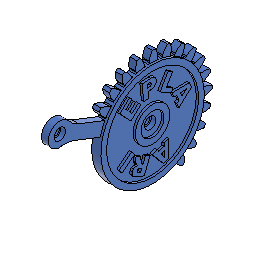
05 Engranaje grande superior (Autodesk Fusion 360 design; units mm, degrees)
Autodesk Fusion 360 part; units mm, degrees
(part 1 of 6)
sketch "Boceto1" plane through (0, 0, 0) normal (0, 0, 1) x (1, 0, 0)
  circle A0 centre (0, 0) radius 22.5
  circle A1 centre (0, 0) radius 0.5
extrude "Extruir1" add sketch "Boceto1" along normal blind 3
sketch "Boceto2" plane through (0, 0, 0) normal (0, 0, 1) x (1, 0, 0)
  spline S0 degree 5 poles (23.4214, -1.8244) (23.4316, -1.8252) (23.4521, -1.8265) (23.4829, -1.8277) (23.524, -1.8279) (23.5754, -1.8262) (23.6269, -1.8231) (23.6784, -1.819) (23.7299, -1.8145) (23.7814, -1.8097) (23.833, -1.8045) (23.8845, -1.7988) (23.9361, -1.7926) (23.9876, -1.7857) (24.0392, -1.7781) (24.0907, -1.7698) (24.1423, -1.761) (24.1939, -1.7518) (24.2454, -1.7421) (24.2969, -1.7321) (24.3485, -1.7216) (24.4, -1.7108) (24.4515, -1.6996) (24.503, -1.6879) (24.5544, -1.6758) (24.6059, -1.6633) (24.6573, -1.6504) (24.7087, -1.6371) (24.7602, -1.6235) (24.8115, -1.6095) (24.8629, -1.5952) (24.9142, -1.5805) (24.9655, -1.5655) (25.0168, -1.5501) (25.0681, -1.5344) (25.1193, -1.5184) (25.1706, -1.502) (25.2217, -1.4853) (25.2729, -1.4683) (25.324, -1.451) (25.3751, -1.4333) (25.4262, -1.4154) (25.4772, -1.3971) (25.5282, -1.3786) (25.5792, -1.3597) (25.6301, -1.3406) (25.6811, -1.3211) (25.7319, -1.3014) (25.7828, -1.2814) (25.8336, -1.2611) (25.8843, -1.2405) (25.935, -1.2196) (25.9857, -1.1985) (26.0364, -1.177) (26.087, -1.1553) (26.1375, -1.1334) (26.1881, -1.1111) (26.2386, -1.0886) (26.289, -1.0658) (26.3394, -1.0428) (26.3897, -1.0194) (26.4401, -0.9959) (26.4903, -0.972) (26.5405, -0.948) (26.5907, -0.9236) (26.6409, -0.899) (26.6909, -0.8742) (26.741, -0.849) (26.791, -0.8237) (26.8409, -0.7981) (26.8908, -0.7722) (26.9307, -0.7514) (26.9605, -0.7356) (26.9805, -0.725) (26.9904, -0.7197) knots 0 0 0 0 0 0 0.01428571 0.02857143 0.04285714 0.05714286 0.07142857 0.08571429 0.1 0.11428571 0.12857143 0.14285714 0.15714286 0.17142857 0.18571429 0.2 0.21428571 0.22857143 0.24285714 0.25714286 0.27142857 0.28571429 0.3 0.31428571 0.32857143 0.34285714 0.35714286 0.37142857 0.38571429 0.4 0.41428571 0.42857143 0.44285714 0.45714286 0.47142857 0.48571429 0.5 0.51428571 0.52857143 0.54285714 0.55714286 0.57142857 0.58571429 0.6 0.61428571 0.62857143 0.64285714 0.65714286 0.67142857 0.68571429 0.7 0.71428571 0.72857143 0.74285714 0.75714286 0.77142857 0.78571429 0.8 0.81428571 0.82857143 0.84285714 0.85714286 0.87142857 0.88571429 0.9 0.91428571 0.92857143 0.94285714 0.95714286 0.97142857 0.98571429 1 1 1 1 1 1
  spline S1 degree 5 poles (23.4214, 1.8244) (23.4316, 1.8252) (23.4521, 1.8265) (23.4829, 1.8277) (23.524, 1.8279) (23.5754, 1.8262) (23.6269, 1.8231) (23.6784, 1.819) (23.7299, 1.8145) (23.7814, 1.8097) (23.833, 1.8045) (23.8845, 1.7988) (23.9361, 1.7926) (23.9876, 1.7857) (24.0392, 1.7781) (24.0907, 1.7698) (24.1423, 1.761) (24.1939, 1.7518) (24.2454, 1.7421) (24.2969, 1.7321) (24.3485, 1.7216) (24.4, 1.7108) (24.4515, 1.6996) (24.503, 1.6879) (24.5544, 1.6758) (24.6059, 1.6633) (24.6573, 1.6504) (24.7087, 1.6371) (24.7602, 1.6235) (24.8115, 1.6095) (24.8629, 1.5952) (24.9142, 1.5805) (24.9655, 1.5655) (25.0168, 1.5501) (25.0681, 1.5344) (25.1193, 1.5184) (25.1706, 1.502) (25.2217, 1.4853) (25.2729, 1.4683) (25.324, 1.451) (25.3751, 1.4333) (25.4262, 1.4154) (25.4772, 1.3971) (25.5282, 1.3786) (25.5792, 1.3597) (25.6301, 1.3406) (25.6811, 1.3211) (25.7319, 1.3014) (25.7828, 1.2814) (25.8336, 1.2611) (25.8843, 1.2405) (25.935, 1.2196) (25.9857, 1.1985) (26.0364, 1.177) (26.087, 1.1553) (26.1375, 1.1334) (26.1881, 1.1111) (26.2386, 1.0886) (26.289, 1.0658) (26.3394, 1.0428) (26.3897, 1.0194) (26.4401, 0.9959) (26.4903, 0.972) (26.5405, 0.948) (26.5907, 0.9236) (26.6409, 0.899) (26.6909, 0.8742) (26.741, 0.849) (26.791, 0.8237) (26.8409, 0.7981) (26.8908, 0.7722) (26.9307, 0.7514) (26.9605, 0.7356) (26.9805, 0.725) (26.9904, 0.7197) knots 0 0 0 0 0 0 0.01428571 0.02857143 0.04285714 0.05714286 0.07142857 0.08571429 0.1 0.11428571 0.12857143 0.14285714 0.15714286 0.17142857 0.18571429 0.2 0.21428571 0.22857143 0.24285714 0.25714286 0.27142857 0.28571429 0.3 0.31428571 0.32857143 0.34285714 0.35714286 0.37142857 0.38571429 0.4 0.41428571 0.42857143 0.44285714 0.45714286 0.47142857 0.48571429 0.5 0.51428571 0.52857143 0.54285714 0.55714286 0.57142857 0.58571429 0.6 0.61428571 0.62857143 0.64285714 0.65714286 0.67142857 0.68571429 0.7 0.71428571 0.72857143 0.74285714 0.75714286 0.77142857 0.78571429 0.8 0.81428571 0.82857143 0.84285714 0.85714286 0.87142857 0.88571429 0.9 0.91428571 0.92857143 0.94285714 0.95714286 0.97142857 0.98571429 1 1 1 1 1 1
  arc A0 (26.9904, -0.7197) -> (26.9904, 0.7197) centre (0, 0) ccw
  line L0 (22.4221, -1.7473) -> (23.4214, -1.8244)
  line L1 (22.4221, 1.7473) -> (23.4214, 1.8244)
  line L2 (22.4221, -1.7473) -> (22.4221, 1.7473)
  point P0 (23.6731, -1.8194)
  point P1 (23.9263, -1.7937)
  point P2 (24.1804, -1.7541)
  point P3 (24.4352, -1.703)
  point P4 (24.6905, -1.6417)
  point P5 (24.9462, -1.5711)
  point P6 (25.2021, -1.4917)
  point P7 (25.458, -1.404)
  point P8 (25.714, -1.3083)
  point P9 (25.9699, -1.205)
  point P10 (26.2255, -1.0944)
  point P11 (26.4809, -0.9765)
  point P12 (26.7359, -0.8515)
  point P13 (23.6731, 1.8194)
  point P14 (23.9263, 1.7937)
  point P15 (24.1804, 1.7541)
  point P16 (24.4352, 1.703)
  point P17 (24.6905, 1.6417)
  point P18 (24.9462, 1.5711)
  point P19 (25.2021, 1.4917)
  point P20 (25.458, 1.404)
  point P21 (25.714, 1.3083)
  point P22 (25.9699, 1.205)
  point P23 (26.2255, 1.0944)
  point P24 (26.4809, 0.9765)
  point P25 (26.7359, 0.8515)
extrude "Extruir2" add sketch "Boceto2" along normal blind 3
fillet "Empalme1" radius 0.5 2 edges at (22.432, -1.7481, 1.5) (22.432, 1.7481, 1.5)
pattern_circular "Patrón C1" count 25 over 360 about axis through (0, 0, 0) along (0, 0, 1) of "Extruir2", "Empalme1"
sketch "Boceto3" plane through (0, 0, 0) normal (0, 0, 1) x (1, 0, 0)
  circle A0 centre (0, 0) radius 25 construction
move_body "Desplazar1" bodies 1 to x (0.998027, 0.062791, 0) y (-0.062791, 0.998027, 0) z (0, 0, 1) at (0, 0, 0)
move_body "Desplazar2" bodies 1 to x (0, 0, -1) y (0, 1, 0) z (1, 0, 0) at (0, 0, 0)
move_body "Desplazar3" bodies 1 to x (1, 0, 0) y (0, 1, 0) z (0, 0, 1) at (0, 79.882, 45)
sketch "Boceto5" plane through (3, 0, 0) normal (1, 0, 0) x (0, 1, 0)
  arc A0 (77.8821, 22.5891) -> (79.0573, 22.5151) centre (79.882, 45) ccw
  arc A1 (79.5389, 22.0084) -> (79.0573, 22.5151) centre (79.039, 22.0155) ccw
  line L0 (79.5389, 22.0084) -> (79.5319, 21.5103)
  spline S0 degree 5 poles (79.5319, 21.5103) (79.5317, 21.5) (79.5317, 21.4795) (79.5324, 21.4487) (79.5348, 21.4076) (79.5397, 21.3564) (79.5461, 21.3053) (79.5533, 21.2541) (79.5611, 21.203) (79.5692, 21.1519) (79.5776, 21.1008) (79.5864, 21.0497) (79.5959, 20.9986) (79.606, 20.9476) (79.6169, 20.8966) (79.6283, 20.8457) (79.6404, 20.7948) (79.6528, 20.7439) (79.6657, 20.6931) (79.679, 20.6423) (79.6926, 20.5915) (79.7067, 20.5408) (79.7211, 20.4901) (79.736, 20.4394) (79.7513, 20.3888) (79.767, 20.3382) (79.7831, 20.2877) (79.7996, 20.2372) (79.8165, 20.1868) (79.8336, 20.1364) (79.8512, 20.086) (79.869, 20.0357) (79.8872, 19.9854) (79.9058, 19.9352) (79.9247, 19.885) (79.9439, 19.8349) (79.9635, 19.7848) (79.9833, 19.7348) (80.0035, 19.6848) (80.024, 19.6348) (80.0448, 19.5849) (80.066, 19.5351) (80.0874, 19.4853) (80.1091, 19.4356) (80.1311, 19.3859) (80.1534, 19.3363) (80.176, 19.2867) (80.1989, 19.2371) (80.2221, 19.1877) (80.2455, 19.1382) (80.2693, 19.0889) (80.2933, 19.0396) (80.3176, 18.9903) (80.3421, 18.9411) (80.367, 18.892) (80.3921, 18.8429) (80.4175, 18.7938) (80.4431, 18.7449) (80.469, 18.696) (80.4952, 18.6471) (80.5216, 18.5983) (80.5483, 18.5496) (80.5752, 18.5009) (80.6024, 18.4523) (80.6299, 18.4038) (80.6576, 18.3553) (80.6855, 18.3068) (80.7137, 18.2585) (80.7422, 18.2102) (80.7709, 18.162) (80.7998, 18.1138) (80.8231, 18.0753) (80.8407, 18.0465) (80.8525, 18.0273) (80.8584, 18.0177) knots 0 0 0 0 0 0 0.01428571 0.02857143 0.04285714 0.05714286 0.07142857 0.08571429 0.1 0.11428571 0.12857143 0.14285714 0.15714286 0.17142857 0.18571429 0.2 0.21428571 0.22857143 0.24285714 0.25714286 0.27142857 0.28571429 0.3 0.31428571 0.32857143 0.34285714 0.35714286 0.37142857 0.38571429 0.4 0.41428571 0.42857143 0.44285714 0.45714286 0.47142857 0.48571429 0.5 0.51428571 0.52857143 0.54285714 0.55714286 0.57142857 0.58571429 0.6 0.61428571 0.62857143 0.64285714 0.65714286 0.67142857 0.68571429 0.7 0.71428571 0.72857143 0.74285714 0.75714286 0.77142857 0.78571429 0.8 0.81428571 0.82857143 0.84285714 0.85714286 0.87142857 0.88571429 0.9 0.91428571 0.92857143 0.94285714 0.95714286 0.97142857 0.98571429 1 1 1 1 1 1
  arc A2 (80.8584, 18.0177) -> (82.2951, 18.108) centre (79.882, 45) ccw
  spline S1 degree 5 poles (82.2951, 18.108) (82.2997, 18.1183) (82.309, 18.1388) (82.3229, 18.1697) (82.3412, 18.2108) (82.3639, 18.2622) (82.3863, 18.3136) (82.4085, 18.3651) (82.4304, 18.4166) (82.452, 18.4682) (82.4734, 18.5197) (82.4946, 18.5713) (82.5155, 18.623) (82.5361, 18.6746) (82.5565, 18.7263) (82.5766, 18.7781) (82.5964, 18.8298) (82.616, 18.8816) (82.6353, 18.9334) (82.6543, 18.9852) (82.6731, 19.037) (82.6916, 19.0889) (82.7098, 19.1408) (82.7277, 19.1927) (82.7453, 19.2447) (82.7627, 19.2966) (82.7798, 19.3486) (82.7966, 19.4006) (82.8131, 19.4526) (82.8293, 19.5046) (82.8452, 19.5566) (82.8608, 19.6087) (82.8761, 19.6608) (82.8911, 19.7129) (82.9058, 19.7649) (82.9202, 19.8171) (82.9343, 19.8692) (82.9481, 19.9213) (82.9615, 19.9734) (82.9746, 20.0256) (82.9874, 20.0777) (82.9999, 20.1299) (83.012, 20.182) (83.0238, 20.2342) (83.0352, 20.2863) (83.0462, 20.3385) (83.057, 20.3906) (83.0674, 20.4428) (83.0774, 20.495) (83.087, 20.5471) (83.0963, 20.5992) (83.1051, 20.6514) (83.1135, 20.7035) (83.1215, 20.7556) (83.1291, 20.8077) (83.1363, 20.8598) (83.1431, 20.9118) (83.1495, 20.9639) (83.1555, 21.0159) (83.161, 21.0679) (83.166, 21.1199) (83.1704, 21.1718) (83.174, 21.2237) (83.177, 21.2756) (83.1794, 21.3274) (83.1814, 21.3791) (83.183, 21.4309) (83.1842, 21.4826) (83.185, 21.5342) (83.1849, 21.5858) (83.1834, 21.6372) (83.1806, 21.6782) (83.1775, 21.7088) (83.1749, 21.7292) (83.1734, 21.7394) knots -1 -1 -1 -1 -1 -1 -0.98571429 -0.97142857 -0.95714286 -0.94285714 -0.92857143 -0.91428571 -0.9 -0.88571429 -0.87142857 -0.85714286 -0.84285714 -0.82857143 -0.81428571 -0.8 -0.78571429 -0.77142857 -0.75714286 -0.74285714 -0.72857143 -0.71428571 -0.7 -0.68571429 -0.67142857 -0.65714286 -0.64285714 -0.62857143 -0.61428571 -0.6 -0.58571429 -0.57142857 -0.55714286 -0.54285714 -0.52857143 -0.51428571 -0.5 -0.48571429 -0.47142857 -0.45714286 -0.44285714 -0.42857143 -0.41428571 -0.4 -0.38571429 -0.37142857 -0.35714286 -0.34285714 -0.32857143 -0.31428571 -0.3 -0.28571429 -0.27142857 -0.25714286 -0.24285714 -0.22857143 -0.21428571 -0.2 -0.18571429 -0.17142857 -0.15714286 -0.14285714 -0.12857143 -0.11428571 -0.1 -0.08571429 -0.07142857 -0.05714286 -0.04285714 -0.02857143 -0.01428571 0 0 0 0 0 0
  line L1 (83.1734, 21.7394) -> (83.104, 22.2327)
  arc A3 (83.5183, 22.7958) -> (83.104, 22.2327) centre (83.5991, 22.3024) ccw
  arc A4 (83.5183, 22.7958) -> (84.675, 23.0164) centre (79.882, 45) ccw
  arc A5 (85.2675, 22.6454) -> (84.675, 23.0164) centre (84.7815, 22.5279) ccw
  line L2 (85.2675, 22.6454) -> (85.3845, 22.1612)
  spline S2 degree 5 poles (85.3845, 22.1612) (85.387, 22.1512) (85.392, 22.1313) (85.4004, 22.1016) (85.4129, 22.0625) (85.4304, 22.0141) (85.4493, 21.9661) (85.469, 21.9184) (85.4892, 21.8708) (85.5098, 21.8233) (85.5306, 21.7759) (85.5519, 21.7286) (85.5738, 21.6815) (85.5963, 21.6346) (85.6195, 21.5879) (85.6432, 21.5414) (85.6675, 21.4951) (85.6923, 21.449) (85.7174, 21.4029) (85.7429, 21.357) (85.7687, 21.3112) (85.7949, 21.2656) (85.8216, 21.2201) (85.8486, 21.1747) (85.876, 21.1295) (85.9038, 21.0844) (85.932, 21.0395) (85.9605, 20.9947) (85.9893, 20.95) (86.0185, 20.9055) (86.048, 20.8611) (86.0778, 20.8168) (86.108, 20.7726) (86.1384, 20.7286) (86.1692, 20.6847) (86.2003, 20.6409) (86.2317, 20.5972) (86.2634, 20.5537) (86.2954, 20.5103) (86.3276, 20.467) (86.3602, 20.4239) (86.393, 20.3809) (86.4262, 20.338) (86.4596, 20.2952) (86.4932, 20.2525) (86.5272, 20.21) (86.5614, 20.1676) (86.5959, 20.1253) (86.6307, 20.0832) (86.6657, 20.0411) (86.7009, 19.9992) (86.7365, 19.9574) (86.7722, 19.9158) (86.8083, 19.8742) (86.8446, 19.8328) (86.8811, 19.7915) (86.9179, 19.7503) (86.9549, 19.7093) (86.9921, 19.6683) (87.0296, 19.6275) (87.0673, 19.5868) (87.1053, 19.5463) (87.1435, 19.5058) (87.1819, 19.4655) (87.2206, 19.4253) (87.2595, 19.3852) (87.2986, 19.3453) (87.3379, 19.3055) (87.3775, 19.2657) (87.4173, 19.2262) (87.4573, 19.1867) (87.4895, 19.1552) (87.5137, 19.1317) (87.5299, 19.116) (87.538, 19.1082) knots 0 0 0 0 0 0 0.01428571 0.02857143 0.04285714 0.05714286 0.07142857 0.08571429 0.1 0.11428571 0.12857143 0.14285714 0.15714286 0.17142857 0.18571429 0.2 0.21428571 0.22857143 0.24285714 0.25714286 0.27142857 0.28571429 0.3 0.31428571 0.32857143 0.34285714 0.35714286 0.37142857 0.38571429 0.4 0.41428571 0.42857143 0.44285714 0.45714286 0.47142857 0.48571429 0.5 0.51428571 0.52857143 0.54285714 0.55714286 0.57142857 0.58571429 0.6 0.61428571 0.62857143 0.64285714 0.65714286 0.67142857 0.68571429 0.7 0.71428571 0.72857143 0.74285714 0.75714286 0.77142857 0.78571429 0.8 0.81428571 0.82857143 0.84285714 0.85714286 0.87142857 0.88571429 0.9 0.91428571 0.92857143 0.94285714 0.95714286 0.97142857 0.98571429 1 1 1 1 1 1
  arc A6 (87.538, 19.1082) -> (88.907, 19.553) centre (79.882, 45) ccw
  spline S3 degree 5 poles (88.907, 19.553) (88.909, 19.5641) (88.9129, 19.5863) (88.9186, 19.6196) (88.9262, 19.664) (88.9353, 19.7194) (88.9443, 19.7748) (88.9529, 19.8302) (88.9613, 19.8855) (88.9695, 19.9408) (88.9774, 19.9961) (88.9851, 20.0514) (88.9924, 20.1066) (88.9996, 20.1618) (89.0064, 20.2169) (89.0131, 20.272) (89.0194, 20.327) (89.0255, 20.382) (89.0313, 20.437) (89.0368, 20.4919) (89.0421, 20.5468) (89.0471, 20.6017) (89.0518, 20.6565) (89.0563, 20.7112) (89.0605, 20.7659) (89.0644, 20.8205) (89.068, 20.8751) (89.0713, 20.9296) (89.0744, 20.9841) (89.0771, 21.0385) (89.0796, 21.0929) (89.0818, 21.1472) (89.0837, 21.2015) (89.0852, 21.2556) (89.0865, 21.3097) (89.0875, 21.3638) (89.0882, 21.4178) (89.0886, 21.4717) (89.0886, 21.5255) (89.0884, 21.5793) (89.0878, 21.633) (89.0869, 21.6866) (89.0856, 21.7401) (89.0841, 21.7936) (89.0822, 21.8469) (89.0799, 21.9002) (89.0773, 21.9534) (89.0744, 22.0065) (89.0711, 22.0595) (89.0675, 22.1124) (89.0635, 22.1652) (89.0591, 22.2179) (89.0543, 22.2705) (89.0491, 22.3229) (89.0435, 22.3753) (89.0375, 22.4275) (89.0311, 22.4796) (89.0244, 22.5316) (89.0173, 22.5835) (89.0097, 22.6353) (89.0016, 22.6868) (88.9929, 22.7382) (88.9835, 22.7894) (88.9735, 22.8404) (88.963, 22.8911) (88.952, 22.9418) (88.9407, 22.9923) (88.929, 23.0427) (88.917, 23.0929) (88.9041, 23.1428) (88.8898, 23.1922) (88.8769, 23.2312) (88.8662, 23.2601) (88.8586, 23.2792) (88.8547, 23.2887) knots -1 -1 -1 -1 -1 -1 -0.98571429 -0.97142857 -0.95714286 -0.94285714 -0.92857143 -0.91428571 -0.9 -0.88571429 -0.87142857 -0.85714286 -0.84285714 -0.82857143 -0.81428571 -0.8 -0.78571429 -0.77142857 -0.75714286 -0.74285714 -0.72857143 -0.71428571 -0.7 -0.68571429 -0.67142857 -0.65714286 -0.64285714 -0.62857143 -0.61428571 -0.6 -0.58571429 -0.57142857 -0.55714286 -0.54285714 -0.52857143 -0.51428571 -0.5 -0.48571429 -0.47142857 -0.45714286 -0.44285714 -0.42857143 -0.41428571 -0.4 -0.38571429 -0.37142857 -0.35714286 -0.34285714 -0.32857143 -0.31428571 -0.3 -0.28571429 -0.27142857 -0.25714286 -0.24285714 -0.22857143 -0.21428571 -0.2 -0.18571429 -0.17142857 -0.15714286 -0.14285714 -0.12857143 -0.11428571 -0.1 -0.08571429 -0.07142857 -0.05714286 -0.04285714 -0.02857143 -0.01428571 0 0 0 0 0 0
  line L3 (88.8547, 23.2887) -> (88.6648, 23.7492)
  arc A7 (88.926, 24.3977) -> (88.6648, 23.7492) centre (89.127, 23.9399) ccw
  arc A8 (88.926, 24.3977) -> (89.9915, 24.899) centre (79.882, 45) ccw
  arc A9 (90.6577, 24.687) -> (89.9915, 24.899) centre (90.2161, 24.4524) ccw
  line L4 (90.6577, 24.687) -> (90.8915, 24.2471)
  spline S4 degree 5 poles (90.8915, 24.2471) (90.8963, 24.2381) (90.9061, 24.22) (90.9216, 24.1934) (90.9434, 24.1586) (90.9724, 24.1161) (91.0027, 24.0743) (91.0336, 24.033) (91.0651, 23.9919) (91.0968, 23.951) (91.1288, 23.9103) (91.1612, 23.8698) (91.194, 23.8296) (91.2275, 23.7898) (91.2616, 23.7503) (91.2961, 23.7112) (91.3312, 23.6724) (91.3667, 23.6338) (91.4024, 23.5955) (91.4385, 23.5573) (91.4749, 23.5194) (91.5117, 23.4817) (91.5488, 23.4443) (91.5862, 23.4071) (91.624, 23.3701) (91.6622, 23.3333) (91.7006, 23.2968) (91.7394, 23.2605) (91.7784, 23.2244) (91.8178, 23.1885) (91.8574, 23.1528) (91.8973, 23.1174) (91.9375, 23.0821) (91.9779, 23.047) (92.0186, 23.0121) (92.0596, 22.9775) (92.1009, 22.943) (92.1424, 22.9087) (92.1842, 22.8746) (92.2262, 22.8408) (92.2685, 22.8071) (92.311, 22.7736) (92.3538, 22.7402) (92.3968, 22.7071) (92.44, 22.6742) (92.4834, 22.6414) (92.5271, 22.6089) (92.5711, 22.5765) (92.6152, 22.5443) (92.6596, 22.5123) (92.7042, 22.4805) (92.749, 22.4488) (92.794, 22.4174) (92.8392, 22.3861) (92.8846, 22.355) (92.9303, 22.3241) (92.9761, 22.2933) (93.0222, 22.2628) (93.0685, 22.2324) (93.1149, 22.2022) (93.1616, 22.1722) (93.2085, 22.1423) (93.2555, 22.1126) (93.3028, 22.0831) (93.3502, 22.0538) (93.3978, 22.0247) (93.4457, 21.9957) (93.4937, 21.9669) (93.5419, 21.9383) (93.5902, 21.9098) (93.6388, 21.8816) (93.6778, 21.8591) (93.7071, 21.8423) (93.7267, 21.8312) (93.7365, 21.8256) knots 0 0 0 0 0 0 0.01428571 0.02857143 0.04285714 0.05714286 0.07142857 0.08571429 0.1 0.11428571 0.12857143 0.14285714 0.15714286 0.17142857 0.18571429 0.2 0.21428571 0.22857143 0.24285714 0.25714286 0.27142857 0.28571429 0.3 0.31428571 0.32857143 0.34285714 0.35714286 0.37142857 0.38571429 0.4 0.41428571 0.42857143 0.44285714 0.45714286 0.47142857 0.48571429 0.5 0.51428571 0.52857143 0.54285714 0.55714286 0.57142857 0.58571429 0.6 0.61428571 0.62857143 0.64285714 0.65714286 0.67142857 0.68571429 0.7 0.71428571 0.72857143 0.74285714 0.75714286 0.77142857 0.78571429 0.8 0.81428571 0.82857143 0.84285714 0.85714286 0.87142857 0.88571429 0.9 0.91428571 0.92857143 0.94285714 0.95714286 0.97142857 0.98571429 1 1 1 1 1 1
  arc A10 (93.7365, 21.8256) -> (94.9519, 22.5969) centre (79.882, 45) ccw
  spline S5 degree 5 poles (94.9519, 22.5969) (94.951, 22.6081) (94.9493, 22.6306) (94.9466, 22.6643) (94.9428, 22.7091) (94.9379, 22.7651) (94.9328, 22.821) (94.9274, 22.8768) (94.9218, 22.9325) (94.916, 22.9881) (94.9099, 23.0436) (94.9035, 23.099) (94.897, 23.1543) (94.8902, 23.2095) (94.8831, 23.2646) (94.8758, 23.3197) (94.8683, 23.3746) (94.8605, 23.4294) (94.8524, 23.484) (94.8441, 23.5386) (94.8356, 23.5931) (94.8268, 23.6475) (94.8178, 23.7017) (94.8085, 23.7558) (94.7989, 23.8098) (94.7891, 23.8637) (94.779, 23.9175) (94.7687, 23.9711) (94.7581, 24.0247) (94.7472, 24.0781) (94.7361, 24.1313) (94.7247, 24.1845) (94.713, 24.2375) (94.7011, 24.2904) (94.6889, 24.3431) (94.6764, 24.3957) (94.6636, 24.4481) (94.6506, 24.5004) (94.6372, 24.5526) (94.6236, 24.6046) (94.6097, 24.6565) (94.5955, 24.7082) (94.581, 24.7597) (94.5662, 24.8111) (94.5511, 24.8623) (94.5356, 24.9133) (94.5199, 24.9642) (94.5039, 25.0149) (94.4875, 25.0654) (94.4709, 25.1158) (94.4539, 25.1659) (94.4365, 25.2159) (94.4188, 25.2656) (94.4007, 25.3151) (94.3822, 25.3644) (94.3634, 25.4135) (94.3443, 25.4624) (94.3248, 25.5111) (94.305, 25.5596) (94.2848, 25.6078) (94.2642, 25.6558) (94.2429, 25.7034) (94.2212, 25.7506) (94.1988, 25.7975) (94.1759, 25.8441) (94.1527, 25.8904) (94.1292, 25.9365) (94.1054, 25.9824) (94.0812, 26.028) (94.0563, 26.0732) (94.0302, 26.1175) (94.008, 26.1521) (93.9905, 26.1774) (93.9783, 26.194) (93.9722, 26.2022) knots -1 -1 -1 -1 -1 -1 -0.98571429 -0.97142857 -0.95714286 -0.94285714 -0.92857143 -0.91428571 -0.9 -0.88571429 -0.87142857 -0.85714286 -0.84285714 -0.82857143 -0.81428571 -0.8 -0.78571429 -0.77142857 -0.75714286 -0.74285714 -0.72857143 -0.71428571 -0.7 -0.68571429 -0.67142857 -0.65714286 -0.64285714 -0.62857143 -0.61428571 -0.6 -0.58571429 -0.57142857 -0.55714286 -0.54285714 -0.52857143 -0.51428571 -0.5 -0.48571429 -0.47142857 -0.45714286 -0.44285714 -0.42857143 -0.41428571 -0.4 -0.38571429 -0.37142857 -0.35714286 -0.34285714 -0.32857143 -0.31428571 -0.3 -0.28571429 -0.27142857 -0.25714286 -0.24285714 -0.22857143 -0.21428571 -0.2 -0.18571429 -0.17142857 -0.15714286 -0.14285714 -0.12857143 -0.11428571 -0.1 -0.08571429 -0.07142857 -0.05714286 -0.04285714 -0.02857143 -0.01428571 0 0 0 0 0 0
  line L5 (93.9722, 26.2022) -> (93.6737, 26.6011)
  arc A11 (93.7655, 27.2941) -> (93.6737, 26.6011) centre (94.074, 26.9006) ccw
  arc A12 (93.7655, 27.2941) -> (94.6728, 28.0447) centre (79.882, 45) ccw
  arc A13 (95.3708, 28.005) -> (94.6728, 28.0447) centre (95.0015, 27.6679) ccw
  line L6 (95.3708, 28.005) -> (95.7066, 27.6371)
  spline S6 degree 5 poles (95.7066, 27.6371) (95.7135, 27.6295) (95.7276, 27.6145) (95.7492, 27.5925) (95.779, 27.5642) (95.8176, 27.5303) (95.8573, 27.4973) (95.8976, 27.465) (95.9382, 27.433) (95.9791, 27.4013) (96.0202, 27.3698) (96.0617, 27.3386) (96.1035, 27.3079) (96.1458, 27.2776) (96.1886, 27.2479) (96.2319, 27.2186) (96.2755, 27.1897) (96.3194, 27.1612) (96.3636, 27.1329) (96.408, 27.105) (96.4527, 27.0773) (96.4977, 27.0499) (96.5429, 27.0229) (96.5885, 26.9962) (96.6343, 26.9697) (96.6803, 26.9436) (96.7267, 26.9178) (96.7733, 26.8923) (96.8201, 26.8671) (96.8671, 26.8421) (96.9143, 26.8174) (96.9618, 26.7929) (97.0095, 26.7687) (97.0574, 26.7448) (97.1055, 26.7212) (97.1538, 26.6978) (97.2024, 26.6747) (97.2511, 26.6518) (97.3001, 26.6292) (97.3492, 26.6068) (97.3985, 26.5847) (97.448, 26.5628) (97.4977, 26.5412) (97.5476, 26.5198) (97.5977, 26.4986) (97.6479, 26.4777) (97.6983, 26.457) (97.7489, 26.4366) (97.7997, 26.4164) (97.8506, 26.3964) (97.9017, 26.3767) (97.953, 26.3572) (98.0044, 26.3379) (98.056, 26.3189) (98.1077, 26.3) (98.1596, 26.2814) (98.2117, 26.2631) (98.2639, 26.2449) (98.3163, 26.227) (98.3688, 26.2093) (98.4215, 26.1918) (98.4743, 26.1746) (98.5272, 26.1575) (98.5803, 26.1407) (98.6336, 26.1241) (98.687, 26.1077) (98.7405, 26.0916) (98.7941, 26.0756) (98.8479, 26.0599) (98.9019, 26.0444) (98.9559, 26.0291) (98.9993, 26.017) (99.0319, 26.008) (99.0536, 26.0021) (99.0645, 25.9991) knots 0 0 0 0 0 0 0.01428571 0.02857143 0.04285714 0.05714286 0.07142857 0.08571429 0.1 0.11428571 0.12857143 0.14285714 0.15714286 0.17142857 0.18571429 0.2 0.21428571 0.22857143 0.24285714 0.25714286 0.27142857 0.28571429 0.3 0.31428571 0.32857143 0.34285714 0.35714286 0.37142857 0.38571429 0.4 0.41428571 0.42857143 0.44285714 0.45714286 0.47142857 0.48571429 0.5 0.51428571 0.52857143 0.54285714 0.55714286 0.57142857 0.58571429 0.6 0.61428571 0.62857143 0.64285714 0.65714286 0.67142857 0.68571429 0.7 0.71428571 0.72857143 0.74285714 0.75714286 0.77142857 0.78571429 0.8 0.81428571 0.82857143 0.84285714 0.85714286 0.87142857 0.88571429 0.9 0.91428571 0.92857143 0.94285714 0.95714286 0.97142857 0.98571429 1 1 1 1 1 1
  arc A14 (99.0645, 25.9991) -> (100.0499, 27.0485) centre (79.882, 45) ccw
  spline S7 degree 5 poles (100.0499, 27.0485) (100.0462, 27.0591) (100.039, 27.0805) (100.028, 27.1124) (100.0132, 27.1549) (99.9945, 27.2079) (99.9756, 27.2608) (99.9566, 27.3135) (99.9373, 27.366) (99.9178, 27.4184) (99.8981, 27.4707) (99.8782, 27.5228) (99.858, 27.5747) (99.8377, 27.6265) (99.8172, 27.6781) (99.7964, 27.7296) (99.7755, 27.7809) (99.7543, 27.832) (99.7329, 27.883) (99.7113, 27.9338) (99.6895, 27.9844) (99.6674, 28.0349) (99.6452, 28.0852) (99.6227, 28.1353) (99.6, 28.1852) (99.5771, 28.235) (99.554, 28.2846) (99.5307, 28.334) (99.5071, 28.3832) (99.4833, 28.4322) (99.4593, 28.481) (99.435, 28.5297) (99.4105, 28.5781) (99.3858, 28.6263) (99.3609, 28.6744) (99.3357, 28.7222) (99.3103, 28.7698) (99.2846, 28.8173) (99.2587, 28.8645) (99.2326, 28.9115) (99.2062, 28.9582) (99.1796, 29.0048) (99.1527, 29.0511) (99.1256, 29.0972) (99.0982, 29.143) (99.0706, 29.1886) (99.0427, 29.234) (99.0146, 29.2791) (98.9862, 29.324) (98.9575, 29.3686) (98.9286, 29.4129) (98.8993, 29.457) (98.8698, 29.5007) (98.84, 29.5442) (98.8098, 29.5873) (98.7794, 29.6302) (98.7487, 29.6728) (98.7177, 29.7152) (98.6865, 29.7572) (98.655, 29.7989) (98.623, 29.8402) (98.5906, 29.8811) (98.5578, 29.9214) (98.5245, 29.9612) (98.4907, 30.0006) (98.4567, 30.0397) (98.4225, 30.0785) (98.388, 30.1171) (98.3533, 30.1553) (98.3179, 30.1928) (98.2816, 30.2292) (98.2515, 30.2572) (98.2282, 30.2774) (98.2123, 30.2904) (98.2043, 30.2969) knots -1 -1 -1 -1 -1 -1 -0.98571429 -0.97142857 -0.95714286 -0.94285714 -0.92857143 -0.91428571 -0.9 -0.88571429 -0.87142857 -0.85714286 -0.84285714 -0.82857143 -0.81428571 -0.8 -0.78571429 -0.77142857 -0.75714286 -0.74285714 -0.72857143 -0.71428571 -0.7 -0.68571429 -0.67142857 -0.65714286 -0.64285714 -0.62857143 -0.61428571 -0.6 -0.58571429 -0.57142857 -0.55714286 -0.54285714 -0.52857143 -0.51428571 -0.5 -0.48571429 -0.47142857 -0.45714286 -0.44285714 -0.42857143 -0.41428571 -0.4 -0.38571429 -0.37142857 -0.35714286 -0.34285714 -0.32857143 -0.31428571 -0.3 -0.28571429 -0.27142857 -0.25714286 -0.24285714 -0.22857143 -0.21428571 -0.2 -0.18571429 -0.17142857 -0.15714286 -0.14285714 -0.12857143 -0.11428571 -0.1 -0.08571429 -0.07142857 -0.05714286 -0.04285714 -0.02857143 -0.01428571 0 0 0 0 0 0
  line L7 (98.2043, 30.2969) -> (97.816, 30.6089)
  arc A15 (97.7326, 31.303) -> (97.816, 30.6089) centre (98.1293, 30.9987) ccw
  arc A16 (97.7326, 31.303) -> (98.4247, 32.2557) centre (79.882, 45) ccw
  arc A17 (99.1106, 32.3908) -> (98.4247, 32.2557) centre (98.8368, 31.9725) ccw
  line L8 (99.1106, 32.3908) -> (99.5274, 32.118)
  spline S8 degree 5 poles (99.5274, 32.118) (99.536, 32.1123) (99.5534, 32.1013) (99.5797, 32.0854) (99.6156, 32.0654) (99.6615, 32.0421) (99.7081, 32.0201) (99.7552, 31.9988) (99.8025, 31.978) (99.85, 31.9574) (99.8977, 31.9371) (99.9456, 31.9172) (99.9938, 31.8978) (100.0423, 31.8791) (100.0911, 31.8609) (100.1403, 31.8433) (100.1897, 31.8261) (100.2393, 31.8094) (100.2892, 31.7931) (100.3392, 31.777) (100.3893, 31.7614) (100.4397, 31.746) (100.4902, 31.7311) (100.541, 31.7165) (100.5919, 31.7023) (100.643, 31.6885) (100.6943, 31.675) (100.7458, 31.6619) (100.7974, 31.6491) (100.8492, 31.6366) (100.9011, 31.6244) (100.9531, 31.6125) (101.0053, 31.6009) (101.0577, 31.5897) (101.1102, 31.5788) (101.1628, 31.5681) (101.2156, 31.5578) (101.2685, 31.5478) (101.3215, 31.538) (101.3746, 31.5286) (101.4279, 31.5194) (101.4813, 31.5105) (101.5348, 31.5019) (101.5884, 31.4936) (101.6422, 31.4856) (101.6961, 31.4778) (101.75, 31.4703) (101.8041, 31.4631) (101.8583, 31.4562) (101.9126, 31.4495) (101.967, 31.4431) (102.0215, 31.4369) (102.0761, 31.4311) (102.1308, 31.4254) (102.1856, 31.4201) (102.2405, 31.415) (102.2955, 31.4101) (102.3506, 31.4055) (102.4058, 31.4012) (102.461, 31.3971) (102.5164, 31.3933) (102.5718, 31.3897) (102.6274, 31.3864) (102.683, 31.3833) (102.7387, 31.3805) (102.7945, 31.3779) (102.8503, 31.3755) (102.9063, 31.3734) (102.9623, 31.3715) (103.0184, 31.3699) (103.0746, 31.3685) (103.1196, 31.3676) (103.1533, 31.3671) (103.1759, 31.3667) (103.1872, 31.3666) knots 0 0 0 0 0 0 0.01428571 0.02857143 0.04285714 0.05714286 0.07142857 0.08571429 0.1 0.11428571 0.12857143 0.14285714 0.15714286 0.17142857 0.18571429 0.2 0.21428571 0.22857143 0.24285714 0.25714286 0.27142857 0.28571429 0.3 0.31428571 0.32857143 0.34285714 0.35714286 0.37142857 0.38571429 0.4 0.41428571 0.42857143 0.44285714 0.45714286 0.47142857 0.48571429 0.5 0.51428571 0.52857143 0.54285714 0.55714286 0.57142857 0.58571429 0.6 0.61428571 0.62857143 0.64285714 0.65714286 0.67142857 0.68571429 0.7 0.71428571 0.72857143 0.74285714 0.75714286 0.77142857 0.78571429 0.8 0.81428571 0.82857143 0.84285714 0.85714286 0.87142857 0.88571429 0.9 0.91428571 0.92857143 0.94285714 0.95714286 0.97142857 0.98571429 1 1 1 1 1 1
  arc A18 (103.1872, 31.3666) -> (103.8806, 32.628) centre (79.882, 45) ccw
  spline S9 degree 5 poles (103.8806, 32.628) (103.8745, 32.6374) (103.8621, 32.6563) (103.8435, 32.6845) (103.8186, 32.722) (103.7874, 32.7687) (103.7559, 32.8152) (103.7243, 32.8615) (103.6926, 32.9076) (103.6607, 32.9535) (103.6286, 32.9992) (103.5964, 33.0447) (103.564, 33.09) (103.5314, 33.1351) (103.4987, 33.18) (103.4658, 33.2247) (103.4327, 33.2692) (103.3995, 33.3134) (103.3661, 33.3575) (103.3325, 33.4013) (103.2988, 33.4449) (103.2649, 33.4883) (103.2308, 33.5315) (103.1966, 33.5745) (103.1622, 33.6172) (103.1277, 33.6597) (103.0929, 33.7019) (103.058, 33.744) (103.023, 33.7858) (102.9877, 33.8273) (102.9523, 33.8687) (102.9167, 33.9097) (102.881, 33.9506) (102.845, 33.9911) (102.8089, 34.0315) (102.7726, 34.0715) (102.7362, 34.1113) (102.6995, 34.1509) (102.6627, 34.1902) (102.6257, 34.2292) (102.5886, 34.2679) (102.5512, 34.3064) (102.5137, 34.3446) (102.4759, 34.3825) (102.438, 34.4201) (102.3999, 34.4574) (102.3616, 34.4944) (102.3231, 34.5311) (102.2845, 34.5675) (102.2456, 34.6036) (102.2065, 34.6393) (102.1673, 34.6747) (102.1278, 34.7098) (102.0881, 34.7444) (102.0481, 34.7787) (102.008, 34.8127) (101.9677, 34.8463) (101.9272, 34.8796) (101.8865, 34.9126) (101.8455, 34.9451) (101.8043, 34.9772) (101.7628, 35.0087) (101.7209, 35.0396) (101.6788, 35.0699) (101.6363, 35.0997) (101.5936, 35.129) (101.5508, 35.1581) (101.5079, 35.1869) (101.4647, 35.2152) (101.4211, 35.2428) (101.3769, 35.2691) (101.3408, 35.2887) (101.3132, 35.3024) (101.2946, 35.3111) (101.2852, 35.3154) knots -1 -1 -1 -1 -1 -1 -0.98571429 -0.97142857 -0.95714286 -0.94285714 -0.92857143 -0.91428571 -0.9 -0.88571429 -0.87142857 -0.85714286 -0.84285714 -0.82857143 -0.81428571 -0.8 -0.78571429 -0.77142857 -0.75714286 -0.74285714 -0.72857143 -0.71428571 -0.7 -0.68571429 -0.67142857 -0.65714286 -0.64285714 -0.62857143 -0.61428571 -0.6 -0.58571429 -0.57142857 -0.55714286 -0.54285714 -0.52857143 -0.51428571 -0.5 -0.48571429 -0.47142857 -0.45714286 -0.44285714 -0.42857143 -0.41428571 -0.4 -0.38571429 -0.37142857 -0.35714286 -0.34285714 -0.32857143 -0.31428571 -0.3 -0.28571429 -0.27142857 -0.25714286 -0.24285714 -0.22857143 -0.21428571 -0.2 -0.18571429 -0.17142857 -0.15714286 -0.14285714 -0.12857143 -0.11428571 -0.1 -0.08571429 -0.07142857 -0.05714286 -0.04285714 -0.02857143 -0.01428571 0 0 0 0 0 0
  line L9 (101.2852, 35.3154) -> (100.8315, 35.5211)
  arc A19 (100.5781, 36.1726) -> (100.8315, 35.5211) centre (101.038, 35.9765) ccw
  arc A20 (100.5781, 36.1726) -> (101.0116, 37.2674) centre (79.882, 45) ccw
  arc A21 (101.6423, 37.5689) -> (101.0116, 37.2674) centre (101.4811, 37.0956) ccw
  line L10 (101.6423, 37.5689) -> (102.1139, 37.4083)
  spline S10 degree 5 poles (102.1139, 37.4083) (102.1236, 37.405) (102.1431, 37.3986) (102.1726, 37.3897) (102.2124, 37.3793) (102.2626, 37.3682) (102.3132, 37.3584) (102.3641, 37.3495) (102.4151, 37.3411) (102.4662, 37.333) (102.5175, 37.3252) (102.5688, 37.3178) (102.6203, 37.311) (102.6719, 37.3049) (102.7238, 37.2995) (102.7758, 37.2946) (102.8279, 37.2903) (102.8801, 37.2865) (102.9325, 37.283) (102.9849, 37.28) (103.0374, 37.2772) (103.09, 37.2749) (103.1426, 37.273) (103.1954, 37.2715) (103.2483, 37.2704) (103.3012, 37.2697) (103.3543, 37.2695) (103.4074, 37.2695) (103.4605, 37.2699) (103.5138, 37.2707) (103.5671, 37.2718) (103.6205, 37.2733) (103.6739, 37.275) (103.7274, 37.2772) (103.781, 37.2796) (103.8346, 37.2824) (103.8883, 37.2855) (103.942, 37.289) (103.9958, 37.2927) (104.0496, 37.2968) (104.1035, 37.3012) (104.1574, 37.3059) (104.2114, 37.3108) (104.2654, 37.3161) (104.3195, 37.3217) (104.3736, 37.3276) (104.4277, 37.3337) (104.4819, 37.3402) (104.5361, 37.347) (104.5903, 37.354) (104.6446, 37.3613) (104.699, 37.3689) (104.7533, 37.3768) (104.8077, 37.385) (104.8621, 37.3934) (104.9165, 37.4021) (104.971, 37.4111) (105.0255, 37.4203) (105.08, 37.4299) (105.1346, 37.4397) (105.1892, 37.4497) (105.2437, 37.46) (105.2984, 37.4706) (105.353, 37.4815) (105.4077, 37.4926) (105.4623, 37.5039) (105.517, 37.5155) (105.5717, 37.5274) (105.6264, 37.5395) (105.6812, 37.5519) (105.7359, 37.5646) (105.7797, 37.5749) (105.8126, 37.5827) (105.8345, 37.588) (105.8455, 37.5906) knots 0 0 0 0 0 0 0.01428571 0.02857143 0.04285714 0.05714286 0.07142857 0.08571429 0.1 0.11428571 0.12857143 0.14285714 0.15714286 0.17142857 0.18571429 0.2 0.21428571 0.22857143 0.24285714 0.25714286 0.27142857 0.28571429 0.3 0.31428571 0.32857143 0.34285714 0.35714286 0.37142857 0.38571429 0.4 0.41428571 0.42857143 0.44285714 0.45714286 0.47142857 0.48571429 0.5 0.51428571 0.52857143 0.54285714 0.55714286 0.57142857 0.58571429 0.6 0.61428571 0.62857143 0.64285714 0.65714286 0.67142857 0.68571429 0.7 0.71428571 0.72857143 0.74285714 0.75714286 0.77142857 0.78571429 0.8 0.81428571 0.82857143 0.84285714 0.85714286 0.87142857 0.88571429 0.9 0.91428571 0.92857143 0.94285714 0.95714286 0.97142857 0.98571429 1 1 1 1 1 1
  arc A22 (105.8455, 37.5906) -> (106.2035, 38.9849) centre (79.882, 45) ccw
  spline S11 degree 5 poles (106.2035, 38.9849) (106.1951, 38.9925) (106.1785, 39.0077) (106.1535, 39.0304) (106.12, 39.0605) (106.0781, 39.098) (106.0361, 39.1352) (105.994, 39.1722) (105.9518, 39.2089) (105.9095, 39.2455) (105.867, 39.2817) (105.8245, 39.3178) (105.7818, 39.3536) (105.7391, 39.3892) (105.6962, 39.4246) (105.6532, 39.4597) (105.6101, 39.4945) (105.567, 39.5291) (105.5237, 39.5635) (105.4803, 39.5976) (105.4367, 39.6315) (105.3931, 39.6651) (105.3494, 39.6984) (105.3056, 39.7315) (105.2616, 39.7643) (105.2176, 39.7969) (105.1734, 39.8292) (105.1292, 39.8612) (105.0848, 39.893) (105.0403, 39.9245) (104.9958, 39.9557) (104.9511, 39.9867) (104.9063, 40.0173) (104.8614, 40.0477) (104.8164, 40.0778) (104.7713, 40.1075) (104.7261, 40.137) (104.6807, 40.1662) (104.6353, 40.1951) (104.5898, 40.2237) (104.5441, 40.252) (104.4984, 40.28) (104.4525, 40.3076) (104.4066, 40.3349) (104.3605, 40.3619) (104.3143, 40.3885) (104.268, 40.4149) (104.2216, 40.4408) (104.1751, 40.4665) (104.1285, 40.4918) (104.0818, 40.5167) (104.0349, 40.5412) (103.988, 40.5653) (103.9409, 40.589) (103.8937, 40.6123) (103.8464, 40.6352) (103.7989, 40.6578) (103.7514, 40.68) (103.7038, 40.7018) (103.656, 40.7231) (103.6082, 40.7439) (103.5601, 40.7641) (103.5119, 40.7836) (103.4635, 40.8025) (103.415, 40.8208) (103.3663, 40.8386) (103.3176, 40.8561) (103.2689, 40.8733) (103.22, 40.89) (103.1709, 40.9059) (103.1216, 40.9203) (103.0817, 40.9303) (103.0516, 40.9368) (103.0314, 40.9406) (103.0213, 40.9424) knots -1 -1 -1 -1 -1 -1 -0.98571429 -0.97142857 -0.95714286 -0.94285714 -0.92857143 -0.91428571 -0.9 -0.88571429 -0.87142857 -0.85714286 -0.84285714 -0.82857143 -0.81428571 -0.8 -0.78571429 -0.77142857 -0.75714286 -0.74285714 -0.72857143 -0.71428571 -0.7 -0.68571429 -0.67142857 -0.65714286 -0.64285714 -0.62857143 -0.61428571 -0.6 -0.58571429 -0.57142857 -0.55714286 -0.54285714 -0.52857143 -0.51428571 -0.5 -0.48571429 -0.47142857 -0.45714286 -0.44285714 -0.42857143 -0.41428571 -0.4 -0.38571429 -0.37142857 -0.35714286 -0.34285714 -0.32857143 -0.31428571 -0.3 -0.28571429 -0.27142857 -0.25714286 -0.24285714 -0.22857143 -0.21428571 -0.2 -0.18571429 -0.17142857 -0.15714286 -0.14285714 -0.12857143 -0.11428571 -0.1 -0.08571429 -0.07142857 -0.05714286 -0.04285714 -0.02857143 -0.01428571 0 0 0 0 0 0
  line L11 (103.0213, 40.9424) -> (102.5307, 41.0288)
  arc A23 (102.1232, 41.5969) -> (102.5307, 41.0288) centre (102.6174, 41.5212) ccw
  arc A24 (102.1232, 41.5969) -> (102.2707, 42.7651) centre (79.882, 45) ccw
  arc A25 (102.8067, 43.2139) -> (102.2707, 42.7651) centre (102.7683, 42.7154) ccw
  line L12 (102.8067, 43.2139) -> (103.3034, 43.1756)
  spline S12 degree 5 poles (103.3034, 43.1756) (103.3136, 43.1748) (103.3342, 43.1735) (103.3649, 43.1723) (103.406, 43.1721) (103.4574, 43.1738) (103.5089, 43.1769) (103.5604, 43.181) (103.6119, 43.1855) (103.6634, 43.1903) (103.715, 43.1955) (103.7665, 43.2012) (103.8181, 43.2074) (103.8696, 43.2143) (103.9212, 43.2219) (103.9728, 43.2302) (104.0243, 43.239) (104.0759, 43.2482) (104.1274, 43.2579) (104.1789, 43.2679) (104.2305, 43.2784) (104.282, 43.2892) (104.3335, 43.3004) (104.385, 43.3121) (104.4364, 43.3242) (104.4879, 43.3367) (104.5393, 43.3496) (104.5908, 43.3629) (104.6422, 43.3765) (104.6935, 43.3905) (104.7449, 43.4048) (104.7962, 43.4195) (104.8476, 43.4345) (104.8989, 43.4499) (104.9501, 43.4656) (105.0014, 43.4816) (105.0526, 43.498) (105.1038, 43.5147) (105.1549, 43.5317) (105.206, 43.549) (105.2571, 43.5667) (105.3082, 43.5846) (105.3592, 43.6029) (105.4103, 43.6214) (105.4612, 43.6403) (105.5122, 43.6594) (105.5631, 43.6789) (105.6139, 43.6986) (105.6648, 43.7186) (105.7156, 43.7389) (105.7663, 43.7595) (105.8171, 43.7804) (105.8677, 43.8015) (105.9184, 43.823) (105.969, 43.8447) (106.0196, 43.8666) (106.0701, 43.8889) (106.1206, 43.9114) (106.171, 43.9342) (106.2214, 43.9572) (106.2718, 43.9806) (106.3221, 44.0041) (106.3723, 44.028) (106.4226, 44.052) (106.4727, 44.0764) (106.5229, 44.101) (106.573, 44.1258) (106.623, 44.151) (106.673, 44.1763) (106.7229, 44.2019) (106.7728, 44.2278) (106.8127, 44.2486) (106.8426, 44.2644) (106.8625, 44.275) (106.8724, 44.2803) knots 0 0 0 0 0 0 0.01428571 0.02857143 0.04285714 0.05714286 0.07142857 0.08571429 0.1 0.11428571 0.12857143 0.14285714 0.15714286 0.17142857 0.18571429 0.2 0.21428571 0.22857143 0.24285714 0.25714286 0.27142857 0.28571429 0.3 0.31428571 0.32857143 0.34285714 0.35714286 0.37142857 0.38571429 0.4 0.41428571 0.42857143 0.44285714 0.45714286 0.47142857 0.48571429 0.5 0.51428571 0.52857143 0.54285714 0.55714286 0.57142857 0.58571429 0.6 0.61428571 0.62857143 0.64285714 0.65714286 0.67142857 0.68571429 0.7 0.71428571 0.72857143 0.74285714 0.75714286 0.77142857 0.78571429 0.8 0.81428571 0.82857143 0.84285714 0.85714286 0.87142857 0.88571429 0.9 0.91428571 0.92857143 0.94285714 0.95714286 0.97142857 0.98571429 1 1 1 1 1 1
  arc A26 (106.8724, 44.2803) -> (106.8724, 45.7197) centre (79.882, 45) ccw
  spline S13 degree 5 poles (106.8724, 45.7197) (106.8625, 45.725) (106.8426, 45.7356) (106.8127, 45.7514) (106.7728, 45.7722) (106.7229, 45.7981) (106.673, 45.8237) (106.623, 45.849) (106.573, 45.8742) (106.5229, 45.899) (106.4727, 45.9236) (106.4226, 45.948) (106.3723, 45.972) (106.3221, 45.9959) (106.2718, 46.0194) (106.2214, 46.0428) (106.171, 46.0658) (106.1206, 46.0886) (106.0701, 46.1111) (106.0196, 46.1334) (105.969, 46.1553) (105.9184, 46.177) (105.8677, 46.1985) (105.8171, 46.2196) (105.7663, 46.2405) (105.7156, 46.2611) (105.6648, 46.2814) (105.6139, 46.3014) (105.5631, 46.3211) (105.5122, 46.3406) (105.4612, 46.3597) (105.4103, 46.3786) (105.3592, 46.3971) (105.3082, 46.4154) (105.2571, 46.4333) (105.206, 46.451) (105.1549, 46.4683) (105.1038, 46.4853) (105.0526, 46.502) (105.0014, 46.5184) (104.9501, 46.5344) (104.8989, 46.5501) (104.8476, 46.5655) (104.7962, 46.5805) (104.7449, 46.5952) (104.6935, 46.6095) (104.6422, 46.6235) (104.5908, 46.6371) (104.5393, 46.6504) (104.4879, 46.6633) (104.4364, 46.6758) (104.385, 46.6879) (104.3335, 46.6996) (104.282, 46.7108) (104.2305, 46.7216) (104.1789, 46.7321) (104.1274, 46.7421) (104.0759, 46.7518) (104.0243, 46.761) (103.9728, 46.7698) (103.9212, 46.7781) (103.8696, 46.7857) (103.8181, 46.7926) (103.7665, 46.7988) (103.715, 46.8045) (103.6634, 46.8097) (103.6119, 46.8145) (103.5604, 46.819) (103.5089, 46.8231) (103.4574, 46.8262) (103.406, 46.8279) (103.3649, 46.8277) (103.3342, 46.8265) (103.3136, 46.8252) (103.3034, 46.8244) knots -1 -1 -1 -1 -1 -1 -0.98571429 -0.97142857 -0.95714286 -0.94285714 -0.92857143 -0.91428571 -0.9 -0.88571429 -0.87142857 -0.85714286 -0.84285714 -0.82857143 -0.81428571 -0.8 -0.78571429 -0.77142857 -0.75714286 -0.74285714 -0.72857143 -0.71428571 -0.7 -0.68571429 -0.67142857 -0.65714286 -0.64285714 -0.62857143 -0.61428571 -0.6 -0.58571429 -0.57142857 -0.55714286 -0.54285714 -0.52857143 -0.51428571 -0.5 -0.48571429 -0.47142857 -0.45714286 -0.44285714 -0.42857143 -0.41428571 -0.4 -0.38571429 -0.37142857 -0.35714286 -0.34285714 -0.32857143 -0.31428571 -0.3 -0.28571429 -0.27142857 -0.25714286 -0.24285714 -0.22857143 -0.21428571 -0.2 -0.18571429 -0.17142857 -0.15714286 -0.14285714 -0.12857143 -0.11428571 -0.1 -0.08571429 -0.07142857 -0.05714286 -0.04285714 -0.02857143 -0.01428571 0 0 0 0 0 0
  line L13 (103.3034, 46.8244) -> (102.8067, 46.7861)
  arc A27 (102.2707, 47.2349) -> (102.8067, 46.7861) centre (102.7683, 47.2846) ccw
  arc A28 (102.2707, 47.2349) -> (102.1232, 48.4031) centre (79.882, 45) ccw
  arc A29 (102.5307, 48.9712) -> (102.1232, 48.4031) centre (102.6174, 48.4788) ccw
  line L14 (102.5307, 48.9712) -> (103.0213, 49.0576)
  spline S14 degree 5 poles (103.0213, 49.0576) (103.0314, 49.0594) (103.0516, 49.0632) (103.0817, 49.0697) (103.1216, 49.0797) (103.1709, 49.0941) (103.22, 49.11) (103.2689, 49.1267) (103.3176, 49.1439) (103.3663, 49.1614) (103.415, 49.1792) (103.4635, 49.1975) (103.5119, 49.2164) (103.5601, 49.2359) (103.6082, 49.2561) (103.656, 49.2769) (103.7038, 49.2982) (103.7514, 49.32) (103.7989, 49.3422) (103.8464, 49.3648) (103.8937, 49.3877) (103.9409, 49.411) (103.988, 49.4347) (104.0349, 49.4588) (104.0818, 49.4833) (104.1285, 49.5082) (104.1751, 49.5335) (104.2216, 49.5592) (104.268, 49.5851) (104.3143, 49.6115) (104.3605, 49.6381) (104.4066, 49.6651) (104.4525, 49.6924) (104.4984, 49.72) (104.5441, 49.748) (104.5898, 49.7763) (104.6353, 49.8049) (104.6807, 49.8338) (104.7261, 49.863) (104.7713, 49.8925) (104.8164, 49.9222) (104.8614, 49.9523) (104.9063, 49.9827) (104.9511, 50.0133) (104.9958, 50.0443) (105.0403, 50.0755) (105.0848, 50.107) (105.1292, 50.1388) (105.1734, 50.1708) (105.2176, 50.2031) (105.2616, 50.2357) (105.3056, 50.2685) (105.3494, 50.3016) (105.3931, 50.3349) (105.4367, 50.3685) (105.4803, 50.4024) (105.5237, 50.4365) (105.567, 50.4709) (105.6101, 50.5055) (105.6532, 50.5403) (105.6962, 50.5754) (105.7391, 50.6108) (105.7818, 50.6464) (105.8245, 50.6822) (105.867, 50.7183) (105.9095, 50.7545) (105.9518, 50.7911) (105.994, 50.8278) (106.0361, 50.8648) (106.0781, 50.902) (106.12, 50.9395) (106.1535, 50.9696) (106.1785, 50.9923) (106.1951, 51.0075) (106.2035, 51.0151) knots 0 0 0 0 0 0 0.01428571 0.02857143 0.04285714 0.05714286 0.07142857 0.08571429 0.1 0.11428571 0.12857143 0.14285714 0.15714286 0.17142857 0.18571429 0.2 0.21428571 0.22857143 0.24285714 0.25714286 0.27142857 0.28571429 0.3 0.31428571 0.32857143 0.34285714 0.35714286 0.37142857 0.38571429 0.4 0.41428571 0.42857143 0.44285714 0.45714286 0.47142857 0.48571429 0.5 0.51428571 0.52857143 0.54285714 0.55714286 0.57142857 0.58571429 0.6 0.61428571 0.62857143 0.64285714 0.65714286 0.67142857 0.68571429 0.7 0.71428571 0.72857143 0.74285714 0.75714286 0.77142857 0.78571429 0.8 0.81428571 0.82857143 0.84285714 0.85714286 0.87142857 0.88571429 0.9 0.91428571 0.92857143 0.94285714 0.95714286 0.97142857 0.98571429 1 1 1 1 1 1
  arc A30 (106.2035, 51.0151) -> (105.8455, 52.4094) centre (79.882, 45) ccw
  spline S15 degree 5 poles (105.8455, 52.4094) (105.8345, 52.412) (105.8126, 52.4173) (105.7797, 52.4251) (105.7359, 52.4354) (105.6812, 52.4481) (105.6264, 52.4605) (105.5717, 52.4726) (105.517, 52.4845) (105.4623, 52.4961) (105.4077, 52.5074) (105.353, 52.5185) (105.2984, 52.5294) (105.2437, 52.54) (105.1892, 52.5503) (105.1346, 52.5603) (105.08, 52.5701) (105.0255, 52.5797) (104.971, 52.5889) (104.9165, 52.5979) (104.8621, 52.6066) (104.8077, 52.615) (104.7533, 52.6232) (104.699, 52.6311) (104.6446, 52.6387) (104.5903, 52.646) (104.5361, 52.653) (104.4819, 52.6598) (104.4277, 52.6663) (104.3736, 52.6724) (104.3195, 52.6783) (104.2654, 52.6839) (104.2114, 52.6892) (104.1574, 52.6941) (104.1035, 52.6988) (104.0496, 52.7032) (103.9958, 52.7073) (103.942, 52.711) (103.8883, 52.7145) (103.8346, 52.7176) (103.781, 52.7204) (103.7274, 52.7228) (103.6739, 52.725) (103.6205, 52.7267) (103.5671, 52.7282) (103.5138, 52.7293) (103.4605, 52.7301) (103.4074, 52.7305) (103.3543, 52.7305) (103.3012, 52.7303) (103.2483, 52.7296) (103.1954, 52.7285) (103.1426, 52.727) (103.09, 52.7251) (103.0374, 52.7228) (102.9849, 52.72) (102.9325, 52.717) (102.8801, 52.7135) (102.8279, 52.7097) (102.7758, 52.7054) (102.7238, 52.7005) (102.6719, 52.6951) (102.6203, 52.689) (102.5688, 52.6822) (102.5175, 52.6748) (102.4662, 52.667) (102.4151, 52.6589) (102.3641, 52.6505) (102.3132, 52.6416) (102.2626, 52.6318) (102.2124, 52.6207) (102.1726, 52.6103) (102.1431, 52.6014) (102.1236, 52.595) (102.1139, 52.5917) knots -1 -1 -1 -1 -1 -1 -0.98571429 -0.97142857 -0.95714286 -0.94285714 -0.92857143 -0.91428571 -0.9 -0.88571429 -0.87142857 -0.85714286 -0.84285714 -0.82857143 -0.81428571 -0.8 -0.78571429 -0.77142857 -0.75714286 -0.74285714 -0.72857143 -0.71428571 -0.7 -0.68571429 -0.67142857 -0.65714286 -0.64285714 -0.62857143 -0.61428571 -0.6 -0.58571429 -0.57142857 -0.55714286 -0.54285714 -0.52857143 -0.51428571 -0.5 -0.48571429 -0.47142857 -0.45714286 -0.44285714 -0.42857143 -0.41428571 -0.4 -0.38571429 -0.37142857 -0.35714286 -0.34285714 -0.32857143 -0.31428571 -0.3 -0.28571429 -0.27142857 -0.25714286 -0.24285714 -0.22857143 -0.21428571 -0.2 -0.18571429 -0.17142857 -0.15714286 -0.14285714 -0.12857143 -0.11428571 -0.1 -0.08571429 -0.07142857 -0.05714286 -0.04285714 -0.02857143 -0.01428571 0 0 0 0 0 0
  line L15 (102.1139, 52.5917) -> (101.6423, 52.4311)
  arc A31 (101.0116, 52.7326) -> (101.6423, 52.4311) centre (101.4811, 52.9044) ccw
  arc A32 (101.0116, 52.7326) -> (100.5781, 53.8274) centre (79.882, 45) ccw
  arc A33 (100.8315, 54.4789) -> (100.5781, 53.8274) centre (101.038, 54.0235) ccw
  line L16 (100.8315, 54.4789) -> (101.2852, 54.6846)
  spline S16 degree 5 poles (101.2852, 54.6846) (101.2946, 54.6889) (101.3132, 54.6976) (101.3408, 54.7113) (101.3769, 54.7309) (101.4211, 54.7572) (101.4647, 54.7848) (101.5079, 54.8131) (101.5508, 54.8419) (101.5936, 54.871) (101.6363, 54.9003) (101.6788, 54.9301) (101.7209, 54.9604) (101.7628, 54.9913) (101.8043, 55.0228) (101.8455, 55.0549) (101.8865, 55.0874) (101.9272, 55.1204) (101.9677, 55.1537) (102.008, 55.1873) (102.0481, 55.2213) (102.0881, 55.2556) (102.1278, 55.2902) (102.1673, 55.3253) (102.2065, 55.3607) (102.2456, 55.3964) (102.2845, 55.4325) (102.3231, 55.4689) (102.3616, 55.5056) (102.3999, 55.5426) (102.438, 55.5799) (102.4759, 55.6175) (102.5137, 55.6554) (102.5512, 55.6936) (102.5886, 55.7321) (102.6257, 55.7708) (102.6627, 55.8098) (102.6995, 55.8491) (102.7362, 55.8887) (102.7726, 55.9285) (102.8089, 55.9685) (102.845, 56.0089) (102.881, 56.0494) (102.9167, 56.0903) (102.9523, 56.1313) (102.9877, 56.1727) (103.023, 56.2142) (103.058, 56.256) (103.0929, 56.2981) (103.1277, 56.3403) (103.1622, 56.3828) (103.1966, 56.4255) (103.2308, 56.4685) (103.2649, 56.5117) (103.2988, 56.5551) (103.3325, 56.5987) (103.3661, 56.6425) (103.3995, 56.6866) (103.4327, 56.7308) (103.4658, 56.7753) (103.4987, 56.82) (103.5314, 56.8649) (103.564, 56.91) (103.5964, 56.9553) (103.6286, 57.0008) (103.6607, 57.0465) (103.6926, 57.0924) (103.7243, 57.1385) (103.7559, 57.1848) (103.7874, 57.2313) (103.8186, 57.278) (103.8435, 57.3155) (103.8621, 57.3437) (103.8745, 57.3626) (103.8806, 57.372) knots 0 0 0 0 0 0 0.01428571 0.02857143 0.04285714 0.05714286 0.07142857 0.08571429 0.1 0.11428571 0.12857143 0.14285714 0.15714286 0.17142857 0.18571429 0.2 0.21428571 0.22857143 0.24285714 0.25714286 0.27142857 0.28571429 0.3 0.31428571 0.32857143 0.34285714 0.35714286 0.37142857 0.38571429 0.4 0.41428571 0.42857143 0.44285714 0.45714286 0.47142857 0.48571429 0.5 0.51428571 0.52857143 0.54285714 0.55714286 0.57142857 0.58571429 0.6 0.61428571 0.62857143 0.64285714 0.65714286 0.67142857 0.68571429 0.7 0.71428571 0.72857143 0.74285714 0.75714286 0.77142857 0.78571429 0.8 0.81428571 0.82857143 0.84285714 0.85714286 0.87142857 0.88571429 0.9 0.91428571 0.92857143 0.94285714 0.95714286 0.97142857 0.98571429 1 1 1 1 1 1
  arc A34 (103.8806, 57.372) -> (103.1872, 58.6334) centre (79.882, 45) ccw